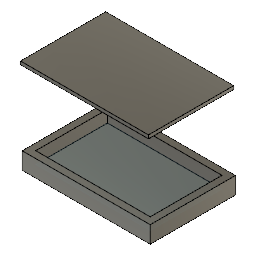
Box attempt 1 v1 (Autodesk Fusion 360 design; units mm, degrees)
Autodesk Fusion 360 part; units mm, degrees
sketch "Sketch1" plane through (0, 0, 0) normal (0, 0, 1) x (1, 0, 0)
  line L0 (0, 0) -> (75, 0)
  line L1 (75, 0) -> (75, 50)
  line L2 (75, 50) -> (0, 50)
  line L3 (0, 50) -> (0, 0)
  line L4 (4, 46) -> (4, 4)
  line L5 (4, 4) -> (71, 4)
  line L6 (71, 4) -> (71, 46)
  line L7 (71, 46) -> (4, 46)
  dimension "d1" = -4
  constraint horizontal L0
  constraint vertical L1
  constraint horizontal L2
  constraint vertical L3
  constraint coincident L0.start L3.end
extrude "Extrude1" add sketch "Sketch1" along normal blind 10 contours L0 L1 L2 L3 | L4 L5 L6 L7 makes body 1
sketch "Sketch2" plane through (0, 0, 10) normal (0, 0, 1) x (-1, 0, 0)
  line L0 (0, -50) -> (0, 0)
  line L1 (0, 0) -> (-75, 0)
  line L2 (-75, 0) -> (-75, -50)
  line L3 (-75, -50) -> (0, -50)
  line L4 (-71, -4) -> (-71, -46)
  line L5 (-71, -46) -> (-4, -46)
  line L6 (-4, -46) -> (-4, -4)
  line L7 (-4, -4) -> (-71, -4)
  dimension "d4" = -4
extrude "Extrude2" cut sketch "Sketch2" against normal blind 7 contours L4 L5 L6 L7 bodies 1
sketch "Sketch3" plane through (0, 0, 3) normal (0, 0, 1) x (-1, 0, 0)
  line L0 (-4, -4) -> (-71, -4)
  line L1 (-71, -4) -> (-71, -46)
  line L2 (-71, -46) -> (-4, -46)
  line L3 (-4, -46) -> (-4, -4)
sketch "Sketch4" plane through (0, 0, 3) normal (0, 0, 1) x (-1, 0, 0)
sketch "Sketch5" plane through (0, 0, 0) normal (0, 0, 1) x (1, 0, 0)
  line L0 (-5, 50) -> (-80, 50)
  line L1 (-80, 50) -> (-80, 0)
  line L2 (-80, 0) -> (-5, 0)
  line L3 (-5, 0) -> (-5, 50)
  line L4 (-75.5, 45.5) -> (-75.5, 4.5)
  line L5 (-75.5, 4.5) -> (-9.5, 4.5)
  line L6 (-9.5, 4.5) -> (-9.5, 45.5)
  line L7 (-9.5, 45.5) -> (-75.5, 45.5)
  dimension "d7" = 75
  dimension "d8" = 50
  dimension "d9" = -4.5
  constraint horizontal L0
  constraint vertical L1
  constraint horizontal L2
  constraint vertical L3
  measures "d7" distance of L0.start L0.end
  measures "d8" distance of L0.start L2.end
extrude "Extrude3" add sketch "Sketch5" along normal blind 2 separate body contours L0 L1 L2 L3 | L4 L5 L6 L7 makes body 2
sketch "Sketch6" plane through (0, 0, 2) normal (0, 0, 1) x (-1, 0, 0)
  line L0 (5, 0) -> (5, -50)
  line L1 (5, -50) -> (80, -50)
  line L2 (80, -50) -> (80, 0)
  line L3 (80, 0) -> (5, 0)
  line L4 (75.5, -45.5) -> (75.5, -4.5)
  line L5 (75.5, -4.5) -> (9.5, -4.5)
  line L6 (9.5, -4.5) -> (9.5, -45.5)
  line L7 (9.5, -45.5) -> (75.5, -45.5)
  dimension "d12" = -4.5
extrude "Extrude4" add sketch "Sketch6" along normal blind 2 contours L4 L5 L6 L7 bodies 2
sketch "Sketch7" plane through (0, 0, 4) normal (0, 0, 1) x (-1, 0, 0)
  line L0 (9.5, -45.5) -> (75.5, -45.5)
  line L1 (75.5, -45.5) -> (75.5, -4.5)
  line L2 (75.5, -4.5) -> (9.5, -4.5)
  line L3 (9.5, -4.5) -> (9.5, -45.5)
  line L4 (73.5, -43.5) -> (73.5, -6.5)
  line L5 (73.5, -6.5) -> (11.5, -6.5)
  line L6 (11.5, -6.5) -> (11.5, -43.5)
  line L7 (11.5, -43.5) -> (73.5, -43.5)
  dimension "d15" = -2
extrude "Extrude5" cut sketch "Sketch7" against normal blind 2 contours L4 L5 L6 L7 bodies 2
copy_body "Body->Comp1" bodies 1 removing the originals makes body 3 in component "Box"
copy_body "Body->Comp2" bodies 2 removing the originals makes body 4 in component "Lid"
move_body "Move1" bodies 4 to x (1, 0, 0) y (0, -1, 0) z (0, 0, -1) at (80, 49, 56) in component "Lid"
component "Box" placed x (1, 0, 0) y (0, 1, 0) z (0, 0, 1) at (0, 0, 0)
component "Lid" placed x (1, 0, 0) y (0, 1, 0) z (0, 0, 1) at (0, 0, 0)
